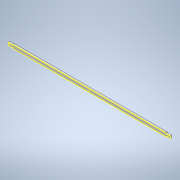
# Autodesk Inventor part: rod_2
Saved by Autodesk Inventor 2022.3 (Build 263350000, 350)
## iProperties
Created: 2023-04-07
Part Number: rod_2
Material: 一般
Document SubType Name: Modeling
Designer: may9c
Density: 1 g/cm^3
Appearance: 預設
Author: may9c
Autodesk Inventor part; units mm, degrees
ref_plane "YZ Plane" through (0, 0, 0) normal (1, 0, 0) x (0, 1, 0)
ref_plane "XZ Plane" through (0, 0, 0) normal (0, 1, 0) x (-1, 0, 0)
ref_plane "XY Plane" through (0, 0, 0) normal (0, 0, 1) x (1, 0, 0)
sketch "草圖1" plane through (0, 0, 0) normal (0, 0, 1) x (1, 0, 0)
  line L0 (-144, 3) -> (0, 3)
  line L1 (0, 3) -> (0, -3)
  line L2 (0, -3) -> (-144, -3)
  line L3 (-144, -3) -> (-144, 3)
  line L4 (-153, 2) -> (-144, 2)
  line L5 (-144, 2) -> (-144, -2)
  line L6 (-144, -2) -> (-153, -2)
  line L7 (-153, -2) -> (-153, 2)
  line L8 (-214.2, 0) -> (214.2, 0) projected
  line L9 (0, -4.2) -> (0, 4.2) projected
  line L10 (144, 3) -> (0, 3)
  line L11 (0, -3) -> (144, -3)
  line L12 (144, -3) -> (144, 3)
  line L13 (153, 2) -> (144, 2)
  line L14 (144, -2) -> (153, -2)
  line L15 (153, -2) -> (153, 2)
  point P0 (0, 0)
  dimension "d0" = 9
  dimension "d1" = 144
  dimension "d2" = 4
  dimension "d3" = 6
  constraints: 28 end point, 6 symmetric about line, 4 parallel, 2 horizontal, 2 perpendicular, 2 point on line, 1 collinear, 2 other
  measures "d0" distance between parallel lines of L7 L3
  measures "d1" distance of L0.start L0.end
  measures "d2" distance between parallel lines of L6 L4
  measures "d3" distance between parallel lines of L2 L0
extrude "擠出1" add sketch "草圖1" along normal blind 3
sketch "草圖2" plane through (0, 0, 3) normal (0, 0, 1) x (1, 0, 0)
  line L0 (-153, -2) -> (-144, -2) projected
  line L1 (-144, -2) -> (-144, -3) projected
  line L2 (-144, -3) -> (144, -3) projected
  line L3 (144, -3) -> (144, -2) projected
  line L4 (144, -2) -> (153, -2) projected
  line L5 (153, -2) -> (153, 2) projected
  line L6 (153, 2) -> (144, 2) projected
  line L7 (144, 2) -> (144, 3) projected
  line L8 (144, 3) -> (-144, 3) projected
  line L9 (-144, 3) -> (-144, 2) projected
  line L10 (-144, 2) -> (-153, 2) projected
  line L11 (-153, 2) -> (-153, -2) projected
  point P0 (0, 0)
